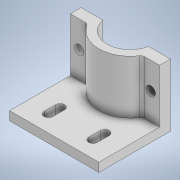
# Autodesk Inventor part: CLAMP
Saved by Autodesk Inventor 2022 (Build 260153000, 153)
## iProperties
Created: 2022-02-10
Part Number: CLAMP
Material: Generic
Document SubType Name: Modeling
Designer: 24sa01
Density: 1 g/cm^3
Appearance: Default
Author: 24sa01
Autodesk Inventor part; units mm, degrees
ref_plane "YZ Plane" through (0, 0, 0) normal (1, 0, 0) x (0, 1, 0)
ref_plane "XZ Plane" through (0, 0, 0) normal (0, 1, 0) x (-1, 0, 0)
ref_plane "XY Plane" through (0, 0, 0) normal (0, 0, 1) x (1, 0, 0)
sketch "Sketch1" plane through (0, 0, 0) normal (0, 1, 0) x (-1, 0, 0)
  line L0 (0, 0) -> (-63.5, 0)
  line L1 (-63.5, 0) -> (-63.5, -50.8)
  line L2 (-63.5, -50.8) -> (0, -50.8)
  line L3 (0, -50.8) -> (0, 0)
  line L4 (-15.875, -11.7475) -> (-15.875, -20.0025) construction
  line L5 (-19.05, -11.7475) -> (-19.05, -20.0025)
  line L6 (-12.7, -20.0025) -> (-12.7, -11.7475)
  arc A0 (-12.7, -11.7475) -> (-19.05, -11.7475) centre (-15.875, -11.7475) ccw
  arc A1 (-19.05, -20.0025) -> (-12.7, -20.0025) centre (-15.875, -20.0025) ccw
  line L7 (-47.625, -11.7475) -> (-47.625, -20.0025) construction
  line L8 (-50.8, -11.7475) -> (-50.8, -20.0025)
  line L9 (-44.45, -20.0025) -> (-44.45, -11.7475)
  arc A2 (-44.45, -11.7475) -> (-50.8, -11.7475) centre (-47.625, -11.7475) ccw
  arc A3 (-50.8, -20.0025) -> (-44.45, -20.0025) centre (-47.625, -20.0025) ccw
  point P0 (-15.875, -15.875)
  point P1 (-47.625, -15.875)
  dimension "d0" = 50.8
  dimension "d1" = 63.5
  dimension "d41" = 8.255
  dimension "d42" = 6.35
  dimension "d43" = 15.875
  dimension "d44" = 8.255
  dimension "d45" = 6.35
  constraints: 24 end point, 8 point on circle, 8 tangent, 4 centre point, 4 parallel, 2 midpoint, 2 vertical, 1 horizontal, 1 perpendicular
  measures "d0" distance of L0.end L1.end
  measures "d1" distance of L1.end L2.end
  measures "d41" distance of L4.start L4.end
  measures "d42" diameter of A1
  measures "d43" distance from line of L3 point (-15.875, -15.875)
  measures "d44" distance of L7.start L7.end
  measures "d45" diameter of A3
extrude "Extrusion1" add sketch "Sketch1" along normal blind 6.35
sketch "Sketch2" plane through (0, 6.35, 0) normal (0, 1, 0) x (1, 0, 0)
  line L0 (63.5, 50.8) -> (0, 50.8)
  circle A0 centre (31.75, 53.975) radius 16.51
  line L1 (0, 50.8) -> (0, 0) projected
  circle A1 centre (31.75, 53.975) radius 22.225
  line L2 (12.3227, 43.18) -> (0, 43.18)
  line L3 (63.5, 50.8) -> (0, 50.8) projected
  line L4 (51.1773, 43.18) -> (63.5, 43.18)
  line L5 (63.5, 0) -> (63.5, 50.8) projected
  point P0 (47.9518, 50.8)
  point P1 (15.5482, 50.8)
  dimension "d22" = 33.02
  dimension "d23" = 3.175
  dimension "d24" = 31.75
  dimension "d25" = 44.45
  dimension "d26" = 7.62
  dimension "d27" = 7.62
  constraints: 6 end point, 2 centre point, 2 point on circle, 2 point on line, 1 coincident, 1 horizontal, 1 perpendicular
  measures "d22" diameter of A0
  measures "d23" distance from line of L0 A0.centre
  measures "d24" distance from line of L1 A0.centre
  measures "d25" diameter of A1
  measures "d26" distance between parallel lines of L0 L2
  measures "d27" distance between parallel lines of L0 L4
extrude "Extrusion2" add sketch "Sketch2" along normal blind 38.1 contours L5 L4 A1 L0 | A1 L0 A0 | L2 L1 L0 A1 picked at (15.4487, 42.02)
sketch "Sketch3" plane through (0, 6.35, -43.18) normal (0, 0, 1) x (1, 0, 0)
  line L0 (63.5, 0) -> (63.5, 38.1) projected
  line L1 (0, 0) -> (0, 38.1) projected
  line L2 (0, 38.1) -> (12.3227, 38.1) projected
  line L3 (51.1773, 38.1) -> (63.5, 38.1) projected
  point P0 (0, -6.35)
  point P1 (6.35, 19.05)
  point P2 (57.15, 19.05)
  dimension "d30" = 6.35
  dimension "d31" = 6.35
  dimension "d32" = 19.05
  dimension "d33" = 19.05
  measures "d30" distance from line of L0 point (57.15, 19.05)
  measures "d31" distance from line of L1 point (6.35, 19.05)
  measures "d32" distance from line of L2 point (6.35, 19.05)
  measures "d33" distance from line of L3 point (57.15, 19.05)
hole "Hole1" at (6.35, 25.4, -43.18) at (57.15, 25.4, -43.18) direction (0, 0, -1) diameter 6.7564 end through all
fillet "Fillet1" radius 3.175 2 edges at (12.3227, 25.4, -43.18) (51.1773, 25.4, -43.18)
body "Solid1"
